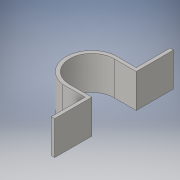
# Autodesk Inventor part: Attachy-thing
Saved by Autodesk Inventor 2016 (Build 200138000, 138)
## iProperties
Created: 2017-01-30
Part Number: Attachy-thing
Material: Generic
Document SubType Name: Modeling
Designer: student1
Density: 1 g/cm^3
Appearance: Default
Author: student1
Autodesk Inventor part; units mm, degrees
ref_plane "YZ Plane" through (0, 0, 0) normal (1, 0, 0) x (0, 1, 0)
ref_plane "XZ Plane" through (0, 0, 0) normal (0, 1, 0) x (-1, 0, 0)
ref_plane "XY Plane" through (0, 0, 0) normal (0, 0, 1) x (1, 0, 0)
sketch "Sketch1" plane through (0, 0, 0) normal (0, 1, 0) x (-1, 0, 0)
  arc A0 (0, -21.6252) -> (0, 11.7758) centre (0, -4.9247) ccw
  line L0 (0, 37.1885) -> (0, 11.7885)
  line L1 (0, -21.6379) -> (0, -47.0379)
  arc A1 (0, -21.6379) -> (0, 11.7885) centre (0, -4.9247) ccw
  line L2 (0, 37.1885) -> (2.54, 37.1885)
  line L3 (0, -47.0379) -> (2.54, -47.0379)
  line L4 (2.54, 37.1885) -> (2.54, 14.3285)
  line L5 (2.54, -47.0379) -> (2.54, -24.1779)
  arc A2 (2.54, -24.1779) -> (2.54, 14.3285) centre (0, -4.9247) ccw
  dimension "d0" = 33.401
  dimension "d1" = 25.4
  dimension "d2" = 25.4
  dimension "d3" = 33.4264
  dimension "d6" = 16.7132
  dimension "d7" = 16.7132
  dimension "d8" = 2.54
  dimension "d9" = 2.54
  dimension "d10" = 19.2532
  dimension "d11" = 19.2532
  constraints: 12 end point, 6 point on circle, 4 vertical, 3 centre point, 2 horizontal, 2 point on line, 1 concentric
  measures "d0" diameter of A0
  measures "d1" distance of L0.start L0.end
  measures "d2" distance of L1.start L1.end
  measures "d3" distance of L1.start L0.end
  measures "d6" distance of L0.end A0.centre
  measures "d7" distance of L1.start A0.centre
  measures "d8" distance of L0.start L2.end
  measures "d9" distance of L1.end L3.end
  measures "d10" vertical distance of L4.end A0.centre
  measures "d11" vertical distance of L5.end A0.centre
extrude "Extrusion1" add sketch "Sketch1" along normal blind 25.4
sketch "Sketch2" plane through (0, 0, 37.1885) normal (1, 0, 0) x (0, 0, -1)
  line L0 (25.4, 0) -> (25.4, 25.4) projected
  line L1 (22.86, 0) -> (22.86, 25.4) projected
  line L2 (25.4, 25.4) -> (22.86, 25.4)
  line L3 (22.86, 25.4) -> (22.86, 0)
  line L4 (22.86, 0) -> (25.4, 0)
  line L5 (25.4, 0) -> (25.4, 25.4)
  line L6 (25.4, 25.4) -> (58.8264, 25.4) projected
  line L7 (61.3664, 0) -> (22.86, 0) projected
  line L8 (58.8264, 25.4) -> (61.3664, 25.4)
  line L9 (61.3664, 25.4) -> (61.3664, 0)
  line L10 (61.3664, 0) -> (58.8264, 0)
  line L11 (58.8264, 0) -> (58.8264, 25.4)
  point P0 (37.1885, 0)
  constraints: 16 end point, 4 parallel, 2 horizontal, 2 perpendicular
extrude "Extrusion2" add sketch "Sketch2" along normal blind 16.7005 contours L4 L1 L2 L0 | L11 L8 L9 L7
sketch "Sketch3" plane through (0, 0, -47.0379) normal (1, 0, 0) x (0, 0, -1)
  line L0 (0, 25.4) -> (-22.86, 25.4) projected
  line L1 (-22.86, 0) -> (0, 0) projected
  line L2 (0, 25.4) -> (-22.86, 25.4)
  line L3 (-22.86, 25.4) -> (-22.86, 0)
  line L4 (-22.86, 0) -> (0, 0)
  line L5 (0, 0) -> (0, 25.4)
  line L6 (-61.3664, 25.4) -> (-84.2264, 25.4) projected
  line L7 (-22.86, 0) -> (-61.3664, 0) projected
  line L8 (-84.2264, 25.4) -> (-61.3664, 25.4)
  line L9 (-61.3664, 25.4) -> (-61.3664, 0)
  line L10 (-61.3664, 0) -> (-84.2264, 0)
  line L11 (-84.2264, 0) -> (-84.2264, 25.4)
  point P0 (-47.0379, 0)
  constraints: 16 end point, 4 parallel, 2 horizontal, 2 perpendicular
extrude "Extrusion3" cut sketch "Sketch3" against normal blind 16.7005
sketch "Sketch4" plane through (16.7005, 25.4, -24.1779) normal (0, 0, -1) x (-1, 0, 0)
  line L0 (0, -25.4) -> (0, 0) projected
  line L1 (16.7005, 0) -> (0, 0) projected
  line L2 (0, -25.4) -> (2.54, -25.4)
  line L3 (2.54, -25.4) -> (2.54, 0)
  line L4 (2.54, 0) -> (0, 0)
  line L5 (0, 0) -> (0, -25.4)
  point P0 (16.7005, -25.4)
  dimension "d18" = 2.54
  constraints: 8 end point, 2 parallel, 1 horizontal, 1 perpendicular, 1 point on line
  measures "d18" distance of L0.start L2.end
extrude "Extrusion4" add sketch "Sketch4" along normal blind 25.4
sketch "Sketch5" plane through (-2.54, 0, 14.3285) normal (0, 0, 1) x (1, 0, 0)
  line L0 (19.2405, 25.4) -> (19.2405, 0) projected
  line L1 (16.7005, 0) -> (16.7005, 25.4) projected
  line L2 (19.2405, 0) -> (16.7005, 0)
  line L3 (16.7005, 0) -> (16.7005, 25.4)
  line L4 (16.7005, 25.4) -> (19.2405, 25.4)
  line L5 (19.2405, 25.4) -> (19.2405, 0)
  point P0 (2.54, 0)
  constraints: 8 end point, 2 parallel, 1 horizontal, 1 perpendicular
extrude "Extrusion5" add sketch "Sketch5" along normal blind 25.4
equation "\"d2\" = d1"
equation "\"d7\" = d6"
equation "\"d9\" = d8"
body "Solid1"
